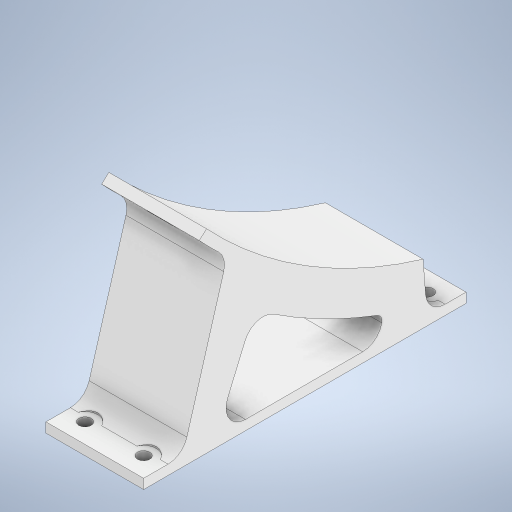
# Autodesk Inventor part: Fuß_Rohr_Aussen
Saved by Autodesk Inventor 2023 (Build 270158000, 158)
## iProperties
Created: 2023-01-04
Part Number: Fuß_Rohr_Aussen
Material: Generisch
Document SubType Name: Modeling
Designer: trist
Density: 1 g/cm^3
Appearance: Weiß
Author: trist
Autodesk Inventor part; units mm, degrees
ref_plane "XZ Plane" through (0, 0, 0) normal (0, 1, 0) x (-1, 0, 0)
sketch "Skizze1" plane through (0, 0, 0) normal (1, 0, 0) x (0, 1, 0)
  line L0 (0, 258) -> (0, -43)
  arc A0 (-170.49959, 182.838425) -> (-239.407602, 72) centre (0, 0) ccw
  line L1 (-270, 50) -> (-270, 215)
  line L2 (-324, 0) -> (54, 0)
  line L3 (-265, 178) -> (-265, 87)
  line L4 (-270, 215) -> (-265, 215)
  line L5 (-265, 215) -> (-265, 195)
  line L6 (0, 0) -> (-170.49959, 182.838425) construction
  arc A1 (-173.909582, 186.495194) -> (-187.990504, 172.292108) centre (0, 0) ccw
  line L7 (-265, 178) -> (-218.731819, 158.292108)
  arc A2 (-218.731819, 158.292108) -> (-253.47781, 93) centre (0, 0) ccw
  line L8 (-239.407602, 72) -> (-265, 70)
  line L9 (-265, 87) -> (-253.47781, 93)
  line L10 (-265, 70) -> (-265, 50)
  line L11 (-265, 50) -> (-270, 50)
  line L12 (-173.909582, 186.495194) -> (-170.49959, 182.838425)
  line L13 (-187.990504, 172.292108) -> (-265, 195)
  dimension "d18" = 250
  dimension "d21" = 270
  dimension "d38" = 5
  dimension "d41" = 5
  dimension "d43" = 20
  dimension "d45" = 17
  dimension "d46" = 17
  dimension "d48" = 215
  dimension "d49" = 20
  dimension "d50" = 20
  dimension "d52" = 21
  dimension "d53" = 14
  dimension "d54" = 270
  dimension "d55" = 50
  dimension "d56" = 72
  dimension "d57" = 47
  dimension "d58" = 255
  constraints: 24 end point, 6 point on circle, 3 centre point, 3 vertical, 2 coincident, 2 perpendicular, 2 point on line, 2 vertical alignment, 1 horizontal
  measures "d18" radius of A0
  measures "d21" distance between parallel lines of L0 L1
  measures "d38" distance between parallel lines of L1 L3
  measures "d41" distance of L6.end L12.start
  measures "d43" distance of L4.end L5.end
  measures "d45" distance of L5.end L3.start
  measures "d46" distance of L3.end L8.end
  measures "d48" distance from line of L2 L1.end
  measures "d49" distance of L8.end L10.end
  measures "d50" distance of L12.start L13.start
  measures "d52" vertical distance of L8.start L9.end
  measures "d53" vertical distance of L7.end L13.start
  measures "d54" radius of A2
  measures "d55" distance from line of L2 L10.end
  measures "d56" distance from line of L2 L8.start
  measures "d57" angle of L2 L6
  measures "d58" radius of A1
extrude "Extrusion2" add sketch "Skizze1" along normal blind 50
fillet "Rundung2" radius 10 6 edges at (25, -265, 195) (25, -265, 178) (25, -187.9905, 172.2921) (25, -218.7318, 158.2921) (25, -265, 87) (25, -265, 70)
fillet "Rundung3" radius 4 1 edges at (25, -253.4778, 93)
ref_plane "Arbeitsebene1" through (10, 0, 0) normal (1, 0, 0) x (0, 1, 0)
sketch "Skizze3" plane through (10, 0, 0) normal (1, 0, 0) x (0, 1, 0)
  line L0 (-265, 215) -> (-270, 215) construction
  line L1 (-265, 202.476972) -> (-265, 215) construction
  line L2 (-270, 215) -> (-270, 50) construction
  line L3 (-265, 202.476972) -> (-265, 215)
  line L4 (-265, 205) -> (-272.989565, 205)
  line L5 (-270, 215) -> (-270, 50)
  line L6 (-270, 205) -> (-270, 208.2)
  line L7 (-270, 208.2) -> (-265, 208.2)
  line L8 (-265, 208.2) -> (-265, 211.5)
  line L9 (-265, 211.5) -> (-255, 211.5)
  line L10 (-255, 211.5) -> (-255, 205)
  line L11 (-255, 205) -> (-270, 205)
  point P0 (0, 0)
  dimension "d62" = 10
  dimension "d63" = 13
  dimension "d64" = 6.4
  dimension "d65" = 10
  constraints: 14 end point, 6 point on line, 3 perpendicular, 1 collinear, 1 horizontal
  measures "d62" distance of L0.start L4.start
  measures "d63" diameter of L9 L4
  measures "d64" diameter of L7 L4
  measures "d65" distance of L8.end L9.end
revolve "Umdrehung1" cut sketch "Skizze3" angle 360 about axis through (10, -265, 205) along (0, -1, 0)
sketch "Skizze4" plane through (10, 0, 0) normal (1, 0, 0) x (0, 1, 0)
  line L0 (-265, 50) -> (-265, 60.750993)
  line L1 (-265, 60) -> (-274.358309, 60)
  line L2 (-270, 215) -> (-270, 50)
  line L3 (-270, 60) -> (-255, 60)
  line L4 (-255, 60) -> (-255, 53.5)
  line L5 (-255, 53.5) -> (-265, 53.5)
  line L6 (-265, 53.5) -> (-265, 56.8)
  line L7 (-265, 56.8) -> (-270, 56.8)
  line L8 (-270, 56.8) -> (-270, 60)
  line L9 (-270, 50) -> (-265, 50)
  point P0 (0, 0)
  point P1 (-267.5, 56.8)
  point P2 (-267.5, 50)
  dimension "d67" = 6.4
  dimension "d68" = 13
  dimension "d69" = 10
  dimension "d70" = 10
  constraints: 14 end point, 6 point on line, 3 perpendicular, 2 horizontal, 2 midpoint
  measures "d67" diameter of point (-267.5, 56.8) L1
  measures "d68" diameter of L5 L1
  measures "d69" distance of L4.end L5.end
  measures "d70" vertical distance of L3.start point (-267.5, 50)
revolve "Umdrehung2" cut sketch "Skizze4" angle 360 about axis through (10, -265, 60) along (0, -1, 0) contours L0 L3 L4 L5 | L7 L2 L1 L0
ref_plane "Arbeitsebene2" through (25, 0, 0) normal (1, 0, 0) x (0, 1, 0)
sketch "Skizze5" plane through (25, 0, 0) normal (1, 0, 0) x (0, 1, 0)
  line L0 (0, 0) -> (-255.486536, 255.486536)
  line L1 (0, 306.583843) -> (0, -51.097307)
  arc A0 (-170.49959, 182.838425) -> (-239.407602, 72) centre (0, 0) ccw
  line L2 (-174.510873, 179.013841) -> (-176.776695, 176.776695)
  line L3 (-187.325708, 187.325708) -> (-182.729514, 191.921902)
  line L4 (-182.729514, 191.921902) -> (-175.70362, 184.805947)
  arc A1 (-173.909582, 186.495194) -> (-183.857462, 176.695879) centre (0, 0) ccw
  line L5 (-175.70362, 184.805947) -> (-178.02389, 182.571889)
  line L6 (-178.02389, 182.571889) -> (-174.510873, 179.013841)
  line L7 (-176.776695, 176.776695) -> (-187.325708, 187.325708)
  point P0 (-176.267381, 180.792865)
  dimension "d72" = 45
  dimension "d73" = 10
  dimension "d74" = 6.4
  dimension "d75" = 13
  constraints: 14 end point, 4 point on circle, 2 perpendicular, 2 point on line, 1 collinear, 1 midpoint, 1 parallel
  measures "d72" angle of L1 L0
  measures "d73" distance of L3.end L4.end
  measures "d74" diameter of point (-176.267, 180.793) L0
  measures "d75" diameter of L3.end L0
revolve "Umdrehung3" cut sketch "Skizze5" angle 360 about axis through (25, 0, 0) along (0, -0.7071068, 0.7071068) contours L0 A1 L6 A0 | L0 L3 L4 A1
pattern_linear "Rechteckige Anordnung1" count 2 spacing 30 along (1, 0, 0) of "Umdrehung1", "Umdrehung2"
sketch "Skizze6" plane through (0, 0, 0) normal (-1, 0, 0) x (0, 0, 1)
  arc A0 (72, -239.407602) -> (182.838425, -170.49959) centre (0, 0) ccw
  circle A1 centre (182.838425, -170.49959) radius 4
  arc A2 (176.695879, -183.857462) -> (186.495194, -173.909582) centre (0, 0) ccw
  circle A3 centre (186.495194, -173.909582) radius 4
  line L0 (70.720596, -255.779107) -> (72, -239.407602)
  circle A4 centre (72, -239.407602) radius 4
  line L1 (50, -270) -> (50, -265)
  circle A5 centre (50, -265) radius 4
  line L2 (215, -270) -> (50, -270)
  circle A6 centre (50, -270) radius 4
  line L3 (215, -265) -> (215, -270)
  circle A7 centre (215, -265) radius 4
  circle A8 centre (215, -270) radius 4
  dimension "d84" = 8
  constraints: 7 centre point, 6 equal radius, 3 coincident
  measures "d84" diameter of A8
